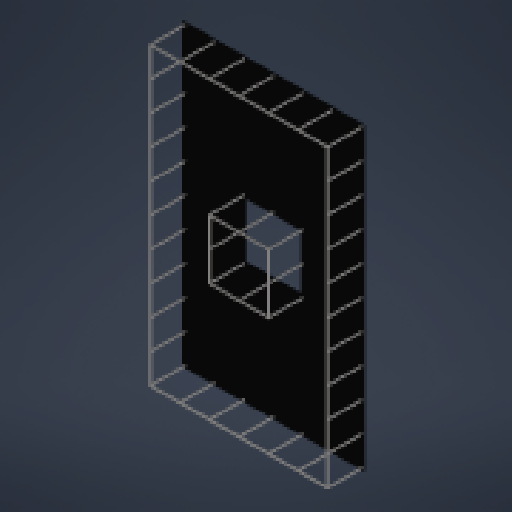
# Autodesk Inventor part: SecondFloor
Saved by Autodesk Inventor 2025 (Build 290162000, 162)
## iProperties
Created: 2024-05-05
Part Number: SecondFloor
Material: Generic
Document SubType Name: Modeling
Designer: zulet
Density: 1 g/cm^3
Appearance: Black
Author: zulet
Autodesk Inventor part; units mm, degrees
(part 1 of 2)
ref_plane "YZ Plane" through (0, 0, 0) normal (1, 0, 0) x (0, 1, 0)
ref_plane "XZ Plane" through (0, 0, 0) normal (0, 1, 0) x (-1, 0, 0)
ref_plane "XY Plane" through (0, 0, 0) normal (0, 0, 1) x (1, 0, 0)
sketch "Sketch1" plane through (0, 0, 0) normal (0, 0, 1) x (1, 0, 0)
  line L0 (183.513924, 6006.538309) -> (183.513924, 4506.538309)
  line L1 (183.513924, 7561.538309) -> (183.513924, 6006.538309)
  line L2 (183.513924, -48.461691) -> (183.513924, 1506.538309)
  line L3 (183.513924, 1506.538309) -> (183.513924, 3006.538309)
  line L4 (183.513924, 4506.538309) -> (183.513924, 3006.538309)
  line L5 (1738.513924, -48.461691) -> (183.513924, -48.461691)
  line L6 (3238.513924, -48.461691) -> (1738.513924, -48.461691)
  line L7 (3238.513924, -48.026006) -> (4793.513924, -48.026006)
  line L8 (4793.513924, -48.461691) -> (4793.513924, 1506.538309)
  line L9 (4793.513924, 3006.538309) -> (4793.513924, 1506.538309)
  line L10 (4793.513924, 3006.538309) -> (4793.513924, 4506.538309)
  line L11 (4793.513924, 4506.538309) -> (4793.513924, 6006.538309)
  line L12 (4793.513924, 7561.538309) -> (4793.513924, 6006.538309)
  line L13 (3238.513924, 7561.538309) -> (4793.513924, 7561.538309)
  line L14 (1738.513924, 7561.973994) -> (3238.513924, 7561.973994)
  line L15 (1738.513924, 7561.538309) -> (183.513924, 7561.538309)
  line L16 (3183.513924, 4561.538309) -> (1793.513924, 4561.538309)
  line L17 (1683.513924, 4451.538309) -> (1683.513924, 3061.538309)
  line L18 (3293.513924, 3061.538309) -> (3293.513924, 4451.538309)
  line L19 (1793.513924, 2951.538309) -> (3183.513924, 2951.538309)
  line L20 (3238.513924, 3006.538309) -> (3183.513924, 2951.538309)
  line L21 (3293.296081, 3061.756152) -> (3238.296081, 3006.756152)
  line L22 (3238.513924, 4506.538309) -> (3183.513924, 4561.538309)
  line L23 (3238.513924, 4506.538309) -> (3293.513924, 4451.538309)
  line L24 (1793.513924, 4561.538309) -> (1738.513924, 4506.538309)
  line L25 (1683.513924, 4451.538309) -> (1738.513924, 4506.538309)
  line L26 (1738.513924, 3006.538309) -> (1683.513924, 3061.538309)
  line L27 (1738.513924, 3006.538309) -> (1793.513924, 2951.538309)
  line L28 (3183.513924, 4451.538309) -> (1793.513924, 4451.538309)
  line L29 (1793.513924, 4451.538309) -> (1793.513924, 3061.538309)
  line L30 (3183.513924, 3061.538309) -> (3183.513924, 4451.538309)
  line L31 (1793.513924, 3061.538309) -> (3183.513924, 3061.538309)
  point P0 (0, 0)
  point P1 (1683.513924, 2185.44858)
  point P2 (1683.513924, 2831.394254)
sketch "Sketch1 outline for Extrusion1" plane through (0, 0, 0) normal (0, 0, 1) x (1, 0, 0)
  line L0 (1738.513924, 7561.538309) -> (183.513924, 7561.538309)
  line L1 (3238.513924, 7561.538309) -> (1738.513924, 7561.538309)
  line L2 (183.513924, 7561.538309) -> (183.513924, 6006.538309)
  line L3 (4793.513924, 7561.538309) -> (3238.513924, 7561.538309)
  line L4 (183.513924, 6006.538309) -> (183.513924, 4506.538309)
  line L5 (4793.513924, 6006.538309) -> (4793.513924, 7561.538309)
  line L6 (183.513924, 4506.538309) -> (183.513924, 3006.538309)
  line L7 (4793.513924, 4506.538309) -> (4793.513924, 6006.538309)
  line L8 (183.513924, 3006.538309) -> (183.513924, 1506.538309)
  line L9 (4793.513924, 3006.538309) -> (4793.513924, 4506.538309)
  line L10 (183.513924, 1506.538309) -> (183.513924, -48.461691)
  line L11 (4793.513924, 1506.538309) -> (4793.513924, 3006.538309)
  line L12 (183.513924, -48.461691) -> (1738.513924, -48.461691)
  line L13 (4793.513924, -48.461691) -> (4793.513924, 1506.538309)
  line L14 (1738.513924, -48.461691) -> (3238.513924, -48.461691)
  line L15 (3238.513924, -48.461691) -> (4793.513924, -48.461691)
  line L16 (3183.513924, 4451.538309) -> (3183.513924, 3061.538309)
  line L17 (1793.513924, 4451.538309) -> (3183.513924, 4451.538309)
  line L18 (1793.513924, 3061.538309) -> (1793.513924, 4451.538309)
  line L19 (3183.513924, 3061.538309) -> (1793.513924, 3061.538309)
extrude "Extrusion1" add sketch "Sketch1 outline for Extrusion1" along normal blind 20
sketch "Sketch2" plane through (0, 0, 20) normal (0, 0, 1) x (1, 0, 0)
  line L0 (231.513924, 7521.538309) -> (255.513924, 7521.538309)
  line L1 (263.513924, 7513.538309) -> (263.513924, 7489.538309)
  line L2 (255.513924, 7481.538309) -> (231.513924, 7481.538309)
  line L3 (223.513924, 7489.538309) -> (223.513924, 7513.538309)
  line L4 (4793.513924, 7561.538309) -> (183.513924, 7561.538309)
  line L5 (183.513924, 7561.538309) -> (183.513924, -48.461691)
  arc A0 (231.513924, 7521.538309) -> (223.513924, 7513.538309) centre (231.513924, 7513.538309) ccw
  arc A1 (263.513924, 7513.538309) -> (255.513924, 7521.538309) centre (255.513924, 7513.538309) ccw
  arc A2 (255.513924, 7481.538309) -> (263.513924, 7489.538309) centre (255.513924, 7489.538309) ccw
  arc A3 (223.513924, 7489.538309) -> (231.513924, 7481.538309) centre (231.513924, 7489.538309) ccw
  line L6 (981.513924, 7521.538309) -> (1005.513924, 7521.538309)
  line L7 (1013.513924, 7513.538309) -> (1013.513924, 7489.538309)
  line L8 (1005.513924, 7481.538309) -> (981.513924, 7481.538309)
  line L9 (973.513924, 7489.538309) -> (973.513924, 7513.538309)
  arc A4 (981.513924, 7521.538309) -> (973.513924, 7513.538309) centre (981.513924, 7513.538309) ccw
  arc A5 (1013.513924, 7513.538309) -> (1005.513924, 7521.538309) centre (1005.513924, 7513.538309) ccw
  arc A6 (1005.513924, 7481.538309) -> (1013.513924, 7489.538309) centre (1005.513924, 7489.538309) ccw
  arc A7 (973.513924, 7489.538309) -> (981.513924, 7481.538309) centre (981.513924, 7489.538309) ccw
  line L10 (1731.513924, 7521.538309) -> (1755.513924, 7521.538309)
  line L11 (1763.513924, 7513.538309) -> (1763.513924, 7489.538309)
  line L12 (1755.513924, 7481.538309) -> (1731.513924, 7481.538309)
  line L13 (1723.513924, 7489.538309) -> (1723.513924, 7513.538309)
  arc A8 (1731.513924, 7521.538309) -> (1723.513924, 7513.538309) centre (1731.513924, 7513.538309) ccw
  arc A9 (1763.513924, 7513.538309) -> (1755.513924, 7521.538309) centre (1755.513924, 7513.538309) ccw
  arc A10 (1755.513924, 7481.538309) -> (1763.513924, 7489.538309) centre (1755.513924, 7489.538309) ccw
  arc A11 (1723.513924, 7489.538309) -> (1731.513924, 7481.538309) centre (1731.513924, 7489.538309) ccw
  line L14 (2481.513924, 7521.538309) -> (2505.513924, 7521.538309)
  line L15 (2513.513924, 7513.538309) -> (2513.513924, 7489.538309)
  line L16 (2505.513924, 7481.538309) -> (2481.513924, 7481.538309)
  line L17 (2473.513924, 7489.538309) -> (2473.513924, 7513.538309)
  arc A12 (2481.513924, 7521.538309) -> (2473.513924, 7513.538309) centre (2481.513924, 7513.538309) ccw
  arc A13 (2513.513924, 7513.538309) -> (2505.513924, 7521.538309) centre (2505.513924, 7513.538309) ccw
  arc A14 (2505.513924, 7481.538309) -> (2513.513924, 7489.538309) centre (2505.513924, 7489.538309) ccw
  arc A15 (2473.513924, 7489.538309) -> (2481.513924, 7481.538309) centre (2481.513924, 7489.538309) ccw
  line L18 (3231.513924, 7521.538309) -> (3255.513924, 7521.538309)
  line L19 (3263.513924, 7513.538309) -> (3263.513924, 7489.538309)
  line L20 (3255.513924, 7481.538309) -> (3231.513924, 7481.538309)
  line L21 (3223.513924, 7489.538309) -> (3223.513924, 7513.538309)
  arc A16 (3231.513924, 7521.538309) -> (3223.513924, 7513.538309) centre (3231.513924, 7513.538309) ccw
  arc A17 (3263.513924, 7513.538309) -> (3255.513924, 7521.538309) centre (3255.513924, 7513.538309) ccw
  arc A18 (3255.513924, 7481.538309) -> (3263.513924, 7489.538309) centre (3255.513924, 7489.538309) ccw
  arc A19 (3223.513924, 7489.538309) -> (3231.513924, 7481.538309) centre (3231.513924, 7489.538309) ccw
  line L22 (3981.513924, 7521.538309) -> (4005.513924, 7521.538309)
  line L23 (4013.513924, 7513.538309) -> (4013.513924, 7489.538309)
  line L24 (4005.513924, 7481.538309) -> (3981.513924, 7481.538309)
  line L25 (3973.513924, 7489.538309) -> (3973.513924, 7513.538309)
  arc A20 (3981.513924, 7521.538309) -> (3973.513924, 7513.538309) centre (3981.513924, 7513.538309) ccw
  arc A21 (4013.513924, 7513.538309) -> (4005.513924, 7521.538309) centre (4005.513924, 7513.538309) ccw
  arc A22 (4005.513924, 7481.538309) -> (4013.513924, 7489.538309) centre (4005.513924, 7489.538309) ccw
  arc A23 (3973.513924, 7489.538309) -> (3981.513924, 7481.538309) centre (3981.513924, 7489.538309) ccw
  line L26 (4731.513924, 7521.538309) -> (4755.513924, 7521.538309)
  line L27 (4763.513924, 7513.538309) -> (4763.513924, 7489.538309)
  line L28 (4755.513924, 7481.538309) -> (4731.513924, 7481.538309)
  line L29 (4723.513924, 7489.538309) -> (4723.513924, 7513.538309)
  arc A24 (4731.513924, 7521.538309) -> (4723.513924, 7513.538309) centre (4731.513924, 7513.538309) ccw
  arc A25 (4763.513924, 7513.538309) -> (4755.513924, 7521.538309) centre (4755.513924, 7513.538309) ccw
  arc A26 (4755.513924, 7481.538309) -> (4763.513924, 7489.538309) centre (4755.513924, 7489.538309) ccw
  arc A27 (4723.513924, 7489.538309) -> (4731.513924, 7481.538309) centre (4731.513924, 7489.538309) ccw
  line L30 (231.513924, 6771.538309) -> (255.513924, 6771.538309)
  line L31 (263.513924, 6763.538309) -> (263.513924, 6739.538309)
  line L32 (255.513924, 6731.538309) -> (231.513924, 6731.538309)
  line L33 (223.513924, 6739.538309) -> (223.513924, 6763.538309)
  arc A28 (231.513924, 6771.538309) -> (223.513924, 6763.538309) centre (231.513924, 6763.538309) ccw
  arc A29 (263.513924, 6763.538309) -> (255.513924, 6771.538309) centre (255.513924, 6763.538309) ccw
  arc A30 (255.513924, 6731.538309) -> (263.513924, 6739.538309) centre (255.513924, 6739.538309) ccw
  arc A31 (223.513924, 6739.538309) -> (231.513924, 6731.538309) centre (231.513924, 6739.538309) ccw
  line L34 (981.513924, 6771.538309) -> (1005.513924, 6771.538309)
  line L35 (1013.513924, 6763.538309) -> (1013.513924, 6739.538309)
  line L36 (1005.513924, 6731.538309) -> (981.513924, 6731.538309)
  line L37 (973.513924, 6739.538309) -> (973.513924, 6763.538309)
  arc A32 (981.513924, 6771.538309) -> (973.513924, 6763.538309) centre (981.513924, 6763.538309) ccw
  arc A33 (1013.513924, 6763.538309) -> (1005.513924, 6771.538309) centre (1005.513924, 6763.538309) ccw
  arc A34 (1005.513924, 6731.538309) -> (1013.513924, 6739.538309) centre (1005.513924, 6739.538309) ccw
  arc A35 (973.513924, 6739.538309) -> (981.513924, 6731.538309) centre (981.513924, 6739.538309) ccw
  line L38 (1731.513924, 6771.538309) -> (1755.513924, 6771.538309)
  line L39 (1763.513924, 6763.538309) -> (1763.513924, 6739.538309)
  line L40 (1755.513924, 6731.538309) -> (1731.513924, 6731.538309)
  line L41 (1723.513924, 6739.538309) -> (1723.513924, 6763.538309)
  arc A36 (1731.513924, 6771.538309) -> (1723.513924, 6763.538309) centre (1731.513924, 6763.538309) ccw
  arc A37 (1763.513924, 6763.538309) -> (1755.513924, 6771.538309) centre (1755.513924, 6763.538309) ccw
  arc A38 (1755.513924, 6731.538309) -> (1763.513924, 6739.538309) centre (1755.513924, 6739.538309) ccw
  arc A39 (1723.513924, 6739.538309) -> (1731.513924, 6731.538309) centre (1731.513924, 6739.538309) ccw
  line L42 (2481.513924, 6771.538309) -> (2505.513924, 6771.538309)
  line L43 (2513.513924, 6763.538309) -> (2513.513924, 6739.538309)
  line L44 (2505.513924, 6731.538309) -> (2481.513924, 6731.538309)
  line L45 (2473.513924, 6739.538309) -> (2473.513924, 6763.538309)
  arc A40 (2481.513924, 6771.538309) -> (2473.513924, 6763.538309) centre (2481.513924, 6763.538309) ccw
  arc A41 (2513.513924, 6763.538309) -> (2505.513924, 6771.538309) centre (2505.513924, 6763.538309) ccw
  arc A42 (2505.513924, 6731.538309) -> (2513.513924, 6739.538309) centre (2505.513924, 6739.538309) ccw
  arc A43 (2473.513924, 6739.538309) -> (2481.513924, 6731.538309) centre (2481.513924, 6739.538309) ccw
  line L46 (3231.513924, 6771.538309) -> (3255.513924, 6771.538309)
  line L47 (3263.513924, 6763.538309) -> (3263.513924, 6739.538309)
  line L48 (3255.513924, 6731.538309) -> (3231.513924, 6731.538309)
  line L49 (3223.513924, 6739.538309) -> (3223.513924, 6763.538309)
  arc A44 (3231.513924, 6771.538309) -> (3223.513924, 6763.538309) centre (3231.513924, 6763.538309) ccw
  arc A45 (3263.513924, 6763.538309) -> (3255.513924, 6771.538309) centre (3255.513924, 6763.538309) ccw
  arc A46 (3255.513924, 6731.538309) -> (3263.513924, 6739.538309) centre (3255.513924, 6739.538309) ccw
  arc A47 (3223.513924, 6739.538309) -> (3231.513924, 6731.538309) centre (3231.513924, 6739.538309) ccw
  line L50 (3981.513924, 6771.538309) -> (4005.513924, 6771.538309)
  line L51 (4013.513924, 6763.538309) -> (4013.513924, 6739.538309)
  line L52 (4005.513924, 6731.538309) -> (3981.513924, 6731.538309)
  line L53 (3973.513924, 6739.538309) -> (3973.513924, 6763.538309)
  arc A48 (3981.513924, 6771.538309) -> (3973.513924, 6763.538309) centre (3981.513924, 6763.538309) ccw
  arc A49 (4013.513924, 6763.538309) -> (4005.513924, 6771.538309) centre (4005.513924, 6763.538309) ccw
  arc A50 (4005.513924, 6731.538309) -> (4013.513924, 6739.538309) centre (4005.513924, 6739.538309) ccw
  arc A51 (3973.513924, 6739.538309) -> (3981.513924, 6731.538309) centre (3981.513924, 6739.538309) ccw
  line L54 (4731.513924, 6771.538309) -> (4755.513924, 6771.538309)
  line L55 (4763.513924, 6763.538309) -> (4763.513924, 6739.538309)
  line L56 (4755.513924, 6731.538309) -> (4731.513924, 6731.538309)
  line L57 (4723.513924, 6739.538309) -> (4723.513924, 6763.538309)
  arc A52 (4731.513924, 6771.538309) -> (4723.513924, 6763.538309) centre (4731.513924, 6763.538309) ccw
  arc A53 (4763.513924, 6763.538309) -> (4755.513924, 6771.538309) centre (4755.513924, 6763.538309) ccw
  arc A54 (4755.513924, 6731.538309) -> (4763.513924, 6739.538309) centre (4755.513924, 6739.538309) ccw
  arc A55 (4723.513924, 6739.538309) -> (4731.513924, 6731.538309) centre (4731.513924, 6739.538309) ccw
  line L58 (231.513924, 6021.538309) -> (255.513924, 6021.538309)
  line L59 (263.513924, 6013.538309) -> (263.513924, 5989.538309)
  line L60 (255.513924, 5981.538309) -> (231.513924, 5981.538309)
  line L61 (223.513924, 5989.538309) -> (223.513924, 6013.538309)
  arc A56 (231.513924, 6021.538309) -> (223.513924, 6013.538309) centre (231.513924, 6013.538309) ccw
  arc A57 (263.513924, 6013.538309) -> (255.513924, 6021.538309) centre (255.513924, 6013.538309) ccw
  arc A58 (255.513924, 5981.538309) -> (263.513924, 5989.538309) centre (255.513924, 5989.538309) ccw
  arc A59 (223.513924, 5989.538309) -> (231.513924, 5981.538309) centre (231.513924, 5989.538309) ccw
  line L62 (981.513924, 6021.538309) -> (1005.513924, 6021.538309)
  line L63 (1013.513924, 6013.538309) -> (1013.513924, 5989.538309)
  line L64 (1005.513924, 5981.538309) -> (981.513924, 5981.538309)
  line L65 (973.513924, 5989.538309) -> (973.513924, 6013.538309)
  arc A60 (981.513924, 6021.538309) -> (973.513924, 6013.538309) centre (981.513924, 6013.538309) ccw
  arc A61 (1013.513924, 6013.538309) -> (1005.513924, 6021.538309) centre (1005.513924, 6013.538309) ccw
  arc A62 (1005.513924, 5981.538309) -> (1013.513924, 5989.538309) centre (1005.513924, 5989.538309) ccw
  arc A63 (973.513924, 5989.538309) -> (981.513924, 5981.538309) centre (981.513924, 5989.538309) ccw
  line L66 (1731.513924, 6021.538309) -> (1755.513924, 6021.538309)
  line L67 (1763.513924, 6013.538309) -> (1763.513924, 5989.538309)
  line L68 (1755.513924, 5981.538309) -> (1731.513924, 5981.538309)
  line L69 (1723.513924, 5989.538309) -> (1723.513924, 6013.538309)
  arc A64 (1731.513924, 6021.538309) -> (1723.513924, 6013.538309) centre (1731.513924, 6013.538309) ccw
  arc A65 (1763.513924, 6013.538309) -> (1755.513924, 6021.538309) centre (1755.513924, 6013.538309) ccw
  arc A66 (1755.513924, 5981.538309) -> (1763.513924, 5989.538309) centre (1755.513924, 5989.538309) ccw
  arc A67 (1723.513924, 5989.538309) -> (1731.513924, 5981.538309) centre (1731.513924, 5989.538309) ccw
  line L70 (2481.513924, 6021.538309) -> (2505.513924, 6021.538309)
  line L71 (2513.513924, 6013.538309) -> (2513.513924, 5989.538309)
  line L72 (2505.513924, 5981.538309) -> (2481.513924, 5981.538309)
  line L73 (2473.513924, 5989.538309) -> (2473.513924, 6013.538309)
  arc A68 (2481.513924, 6021.538309) -> (2473.513924, 6013.538309) centre (2481.513924, 6013.538309) ccw
  arc A69 (2513.513924, 6013.538309) -> (2505.513924, 6021.538309) centre (2505.513924, 6013.538309) ccw
  arc A70 (2505.513924, 5981.538309) -> (2513.513924, 5989.538309) centre (2505.513924, 5989.538309) ccw
  arc A71 (2473.513924, 5989.538309) -> (2481.513924, 5981.538309) centre (2481.513924, 5989.538309) ccw
  line L74 (3231.513924, 6021.538309) -> (3255.513924, 6021.538309)
  line L75 (3263.513924, 6013.538309) -> (3263.513924, 5989.538309)
  line L76 (3255.513924, 5981.538309) -> (3231.513924, 5981.538309)
  line L77 (3223.513924, 5989.538309) -> (3223.513924, 6013.538309)
  arc A72 (3231.513924, 6021.538309) -> (3223.513924, 6013.538309) centre (3231.513924, 6013.538309) ccw
  arc A73 (3263.513924, 6013.538309) -> (3255.513924, 6021.538309) centre (3255.513924, 6013.538309) ccw
  arc A74 (3255.513924, 5981.538309) -> (3263.513924, 5989.538309) centre (3255.513924, 5989.538309) ccw
  arc A75 (3223.513924, 5989.538309) -> (3231.513924, 5981.538309) centre (3231.513924, 5989.538309) ccw
  line L78 (3981.513924, 6021.538309) -> (4005.513924, 6021.538309)
  line L79 (4013.513924, 6013.538309) -> (4013.513924, 5989.538309)
  line L80 (4005.513924, 5981.538309) -> (3981.513924, 5981.538309)
  line L81 (3973.513924, 5989.538309) -> (3973.513924, 6013.538309)
  arc A76 (3981.513924, 6021.538309) -> (3973.513924, 6013.538309) centre (3981.513924, 6013.538309) ccw
  arc A77 (4013.513924, 6013.538309) -> (4005.513924, 6021.538309) centre (4005.513924, 6013.538309) ccw
  arc A78 (4005.513924, 5981.538309) -> (4013.513924, 5989.538309) centre (4005.513924, 5989.538309) ccw
  arc A79 (3973.513924, 5989.538309) -> (3981.513924, 5981.538309) centre (3981.513924, 5989.538309) ccw
  line L82 (4731.513924, 6021.538309) -> (4755.513924, 6021.538309)
  line L83 (4763.513924, 6013.538309) -> (4763.513924, 5989.538309)
  line L84 (4755.513924, 5981.538309) -> (4731.513924, 5981.538309)
  line L85 (4723.513924, 5989.538309) -> (4723.513924, 6013.538309)
  arc A80 (4731.513924, 6021.538309) -> (4723.513924, 6013.538309) centre (4731.513924, 6013.538309) ccw
  arc A81 (4763.513924, 6013.538309) -> (4755.513924, 6021.538309) centre (4755.513924, 6013.538309) ccw
  arc A82 (4755.513924, 5981.538309) -> (4763.513924, 5989.538309) centre (4755.513924, 5989.538309) ccw
  arc A83 (4723.513924, 5989.538309) -> (4731.513924, 5981.538309) centre (4731.513924, 5989.538309) ccw
  line L86 (231.513924, 5271.538309) -> (255.513924, 5271.538309)
  line L87 (263.513924, 5263.538309) -> (263.513924, 5239.538309)
  line L88 (255.513924, 5231.538309) -> (231.513924, 5231.538309)
  line L89 (223.513924, 5239.538309) -> (223.513924, 5263.538309)
  arc A84 (231.513924, 5271.538309) -> (223.513924, 5263.538309) centre (231.513924, 5263.538309) ccw
  arc A85 (263.513924, 5263.538309) -> (255.513924, 5271.538309) centre (255.513924, 5263.538309) ccw
  arc A86 (255.513924, 5231.538309) -> (263.513924, 5239.538309) centre (255.513924, 5239.538309) ccw
  arc A87 (223.513924, 5239.538309) -> (231.513924, 5231.538309) centre (231.513924, 5239.538309) ccw
  line L90 (981.513924, 5271.538309) -> (1005.513924, 5271.538309)
  line L91 (1013.513924, 5263.538309) -> (1013.513924, 5239.538309)
  line L92 (1005.513924, 5231.538309) -> (981.513924, 5231.538309)
  line L93 (973.513924, 5239.538309) -> (973.513924, 5263.538309)
  arc A88 (981.513924, 5271.538309) -> (973.513924, 5263.538309) centre (981.513924, 5263.538309) ccw
  arc A89 (1013.513924, 5263.538309) -> (1005.513924, 5271.538309) centre (1005.513924, 5263.538309) ccw
  arc A90 (1005.513924, 5231.538309) -> (1013.513924, 5239.538309) centre (1005.513924, 5239.538309) ccw
  arc A91 (973.513924, 5239.538309) -> (981.513924, 5231.538309) centre (981.513924, 5239.538309) ccw
  line L94 (1731.513924, 5271.538309) -> (1755.513924, 5271.538309)
  line L95 (1763.513924, 5263.538309) -> (1763.513924, 5239.538309)
  line L96 (1755.513924, 5231.538309) -> (1731.513924, 5231.538309)
  line L97 (1723.513924, 5239.538309) -> (1723.513924, 5263.538309)
  arc A92 (1731.513924, 5271.538309) -> (1723.513924, 5263.538309) centre (1731.513924, 5263.538309) ccw
  arc A93 (1763.513924, 5263.538309) -> (1755.513924, 5271.538309) centre (1755.513924, 5263.538309) ccw
  arc A94 (1755.513924, 5231.538309) -> (1763.513924, 5239.538309) centre (1755.513924, 5239.538309) ccw
  arc A95 (1723.513924, 5239.538309) -> (1731.513924, 5231.538309) centre (1731.513924, 5239.538309) ccw
  line L98 (2481.513924, 5271.538309) -> (2505.513924, 5271.538309)
  line L99 (2513.513924, 5263.538309) -> (2513.513924, 5239.538309)
  line L100 (2505.513924, 5231.538309) -> (2481.513924, 5231.538309)
  line L101 (2473.513924, 5239.538309) -> (2473.513924, 5263.538309)
  arc A96 (2481.513924, 5271.538309) -> (2473.513924, 5263.538309) centre (2481.513924, 5263.538309) ccw
  arc A97 (2513.513924, 5263.538309) -> (2505.513924, 5271.538309) centre (2505.513924, 5263.538309) ccw
  arc A98 (2505.513924, 5231.538309) -> (2513.513924, 5239.538309) centre (2505.513924, 5239.538309) ccw
  arc A99 (2473.513924, 5239.538309) -> (2481.513924, 5231.538309) centre (2481.513924, 5239.538309) ccw
  line L102 (3231.513924, 5271.538309) -> (3255.513924, 5271.538309)
  line L103 (3263.513924, 5263.538309) -> (3263.513924, 5239.538309)
  line L104 (3255.513924, 5231.538309) -> (3231.513924, 5231.538309)
  line L105 (3223.513924, 5239.538309) -> (3223.513924, 5263.538309)
  arc A100 (3231.513924, 5271.538309) -> (3223.513924, 5263.538309) centre (3231.513924, 5263.538309) ccw
  arc A101 (3263.513924, 5263.538309) -> (3255.513924, 5271.538309) centre (3255.513924, 5263.538309) ccw
  arc A102 (3255.513924, 5231.538309) -> (3263.513924, 5239.538309) centre (3255.513924, 5239.538309) ccw
  arc A103 (3223.513924, 5239.538309) -> (3231.513924, 5231.538309) centre (3231.513924, 5239.538309) ccw
  line L106 (3981.513924, 5271.538309) -> (4005.513924, 5271.538309)
  line L107 (4013.513924, 5263.538309) -> (4013.513924, 5239.538309)
  line L108 (4005.513924, 5231.538309) -> (3981.513924, 5231.538309)
  line L109 (3973.513924, 5239.538309) -> (3973.513924, 5263.538309)
  arc A104 (3981.513924, 5271.538309) -> (3973.513924, 5263.538309) centre (3981.513924, 5263.538309) ccw
  arc A105 (4013.513924, 5263.538309) -> (4005.513924, 5271.538309) centre (4005.513924, 5263.538309) ccw
  arc A106 (4005.513924, 5231.538309) -> (4013.513924, 5239.538309) centre (4005.513924, 5239.538309) ccw
  arc A107 (3973.513924, 5239.538309) -> (3981.513924, 5231.538309) centre (3981.513924, 5239.538309) ccw
  line L110 (4731.513924, 5271.538309) -> (4755.513924, 5271.538309)
  line L111 (4763.513924, 5263.538309) -> (4763.513924, 5239.538309)
  line L112 (4755.513924, 5231.538309) -> (4731.513924, 5231.538309)
  line L113 (4723.513924, 5239.538309) -> (4723.513924, 5263.538309)
  arc A108 (4731.513924, 5271.538309) -> (4723.513924, 5263.538309) centre (4731.513924, 5263.538309) ccw
  arc A109 (4763.513924, 5263.538309) -> (4755.513924, 5271.538309) centre (4755.513924, 5263.538309) ccw
  arc A110 (4755.513924, 5231.538309) -> (4763.513924, 5239.538309) centre (4755.513924, 5239.538309) ccw
  arc A111 (4723.513924, 5239.538309) -> (4731.513924, 5231.538309) centre (4731.513924, 5239.538309) ccw
  line L114 (231.513924, 4521.538309) -> (255.513924, 4521.538309)
  line L115 (263.513924, 4513.538309) -> (263.513924, 4489.538309)
  line L116 (255.513924, 4481.538309) -> (231.513924, 4481.538309)
  line L117 (223.513924, 4489.538309) -> (223.513924, 4513.538309)
  arc A112 (231.513924, 4521.538309) -> (223.513924, 4513.538309) centre (231.513924, 4513.538309) ccw
  arc A113 (263.513924, 4513.538309) -> (255.513924, 4521.538309) centre (255.513924, 4513.538309) ccw
  arc A114 (255.513924, 4481.538309) -> (263.513924, 4489.538309) centre (255.513924, 4489.538309) ccw
  arc A115 (223.513924, 4489.538309) -> (231.513924, 4481.538309) centre (231.513924, 4489.538309) ccw
  line L118 (981.513924, 4521.538309) -> (1005.513924, 4521.538309)
  line L119 (1013.513924, 4513.538309) -> (1013.513924, 4489.538309)
  line L120 (1005.513924, 4481.538309) -> (981.513924, 4481.538309)
  line L121 (973.513924, 4489.538309) -> (973.513924, 4513.538309)
  arc A116 (981.513924, 4521.538309) -> (973.513924, 4513.538309) centre (981.513924, 4513.538309) ccw
  arc A117 (1013.513924, 4513.538309) -> (1005.513924, 4521.538309) centre (1005.513924, 4513.538309) ccw
  arc A118 (1005.513924, 4481.538309) -> (1013.513924, 4489.538309) centre (1005.513924, 4489.538309) ccw
  arc A119 (973.513924, 4489.538309) -> (981.513924, 4481.538309) centre (981.513924, 4489.538309) ccw
  line L122 (1731.513924, 4521.538309) -> (1755.513924, 4521.538309)
  line L123 (1763.513924, 4513.538309) -> (1763.513924, 4489.538309)
  line L124 (1755.513924, 4481.538309) -> (1731.513924, 4481.538309)
  line L125 (1723.513924, 4489.538309) -> (1723.513924, 4513.538309)
  arc A120 (1731.513924, 4521.538309) -> (1723.513924, 4513.538309) centre (1731.513924, 4513.538309) ccw
  arc A121 (1763.513924, 4513.538309) -> (1755.513924, 4521.538309) centre (1755.513924, 4513.538309) ccw
  arc A122 (1755.513924, 4481.538309) -> (1763.513924, 4489.538309) centre (1755.513924, 4489.538309) ccw
  arc A123 (1723.513924, 4489.538309) -> (1731.513924, 4481.538309) centre (1731.513924, 4489.538309) ccw
  line L126 (2481.513924, 4521.538309) -> (2505.513924, 4521.538309)
  line L127 (2513.513924, 4513.538309) -> (2513.513924, 4489.538309)
  line L128 (2505.513924, 4481.538309) -> (2481.513924, 4481.538309)
  line L129 (2473.513924, 4489.538309) -> (2473.513924, 4513.538309)
  arc A124 (2481.513924, 4521.538309) -> (2473.513924, 4513.538309) centre (2481.513924, 4513.538309) ccw
  arc A125 (2513.513924, 4513.538309) -> (2505.513924, 4521.538309) centre (2505.513924, 4513.538309) ccw
  arc A126 (2505.513924, 4481.538309) -> (2513.513924, 4489.538309) centre (2505.513924, 4489.538309) ccw
  arc A127 (2473.513924, 4489.538309) -> (2481.513924, 4481.538309) centre (2481.513924, 4489.538309) ccw
  line L130 (3231.513924, 4521.538309) -> (3255.513924, 4521.538309)
  line L131 (3263.513924, 4513.538309) -> (3263.513924, 4489.538309)
  line L132 (3255.513924, 4481.538309) -> (3231.513924, 4481.538309)
  line L133 (3223.513924, 4489.538309) -> (3223.513924, 4513.538309)
  arc A128 (3231.513924, 4521.538309) -> (3223.513924, 4513.538309) centre (3231.513924, 4513.538309) ccw
  arc A129 (3263.513924, 4513.538309) -> (3255.513924, 4521.538309) centre (3255.513924, 4513.538309) ccw
  arc A130 (3255.513924, 4481.538309) -> (3263.513924, 4489.538309) centre (3255.513924, 4489.538309) ccw
  arc A131 (3223.513924, 4489.538309) -> (3231.513924, 4481.538309) centre (3231.513924, 4489.538309) ccw
  line L134 (3981.513924, 4521.538309) -> (4005.513924, 4521.538309)
  line L135 (4013.513924, 4513.538309) -> (4013.513924, 4489.538309)
  line L136 (4005.513924, 4481.538309) -> (3981.513924, 4481.538309)
  line L137 (3973.513924, 4489.538309) -> (3973.513924, 4513.538309)
  arc A132 (3981.513924, 4521.538309) -> (3973.513924, 4513.538309) centre (3981.513924, 4513.538309) ccw
  arc A133 (4013.513924, 4513.538309) -> (4005.513924, 4521.538309) centre (4005.513924, 4513.538309) ccw
  arc A134 (4005.513924, 4481.538309) -> (4013.513924, 4489.538309) centre (4005.513924, 4489.538309) ccw
  arc A135 (3973.513924, 4489.538309) -> (3981.513924, 4481.538309) centre (3981.513924, 4489.538309) ccw
  line L138 (4731.513924, 4521.538309) -> (4755.513924, 4521.538309)
  line L139 (4763.513924, 4513.538309) -> (4763.513924, 4489.538309)
  line L140 (4755.513924, 4481.538309) -> (4731.513924, 4481.538309)
  line L141 (4723.513924, 4489.538309) -> (4723.513924, 4513.538309)
  arc A136 (4731.513924, 4521.538309) -> (4723.513924, 4513.538309) centre (4731.513924, 4513.538309) ccw
  arc A137 (4763.513924, 4513.538309) -> (4755.513924, 4521.538309) centre (4755.513924, 4513.538309) ccw
  arc A138 (4755.513924, 4481.538309) -> (4763.513924, 4489.538309) centre (4755.513924, 4489.538309) ccw
  arc A139 (4723.513924, 4489.538309) -> (4731.513924, 4481.538309) centre (4731.513924, 4489.538309) ccw
  line L142 (231.513924, 3771.538309) -> (255.513924, 3771.538309)
  line L143 (263.513924, 3763.538309) -> (263.513924, 3739.538309)
  line L144 (255.513924, 3731.538309) -> (231.513924, 3731.538309)
  line L145 (223.513924, 3739.538309) -> (223.513924, 3763.538309)
  arc A140 (231.513924, 3771.538309) -> (223.513924, 3763.538309) centre (231.513924, 3763.538309) ccw
  arc A141 (263.513924, 3763.538309) -> (255.513924, 3771.538309) centre (255.513924, 3763.538309) ccw
  arc A142 (255.513924, 3731.538309) -> (263.513924, 3739.538309) centre (255.513924, 3739.538309) ccw
  arc A143 (223.513924, 3739.538309) -> (231.513924, 3731.538309) centre (231.513924, 3739.538309) ccw
  line L146 (981.513924, 3771.538309) -> (1005.513924, 3771.538309)
  line L147 (1013.513924, 3763.538309) -> (1013.513924, 3739.538309)
  line L148 (1005.513924, 3731.538309) -> (981.513924, 3731.538309)
  line L149 (973.513924, 3739.538309) -> (973.513924, 3763.538309)
  arc A144 (981.513924, 3771.538309) -> (973.513924, 3763.538309) centre (981.513924, 3763.538309) ccw
  arc A145 (1013.513924, 3763.538309) -> (1005.513924, 3771.538309) centre (1005.513924, 3763.538309) ccw
  arc A146 (1005.513924, 3731.538309) -> (1013.513924, 3739.538309) centre (1005.513924, 3739.538309) ccw
  arc A147 (973.513924, 3739.538309) -> (981.513924, 3731.538309) centre (981.513924, 3739.538309) ccw
  line L150 (1731.513924, 3771.538309) -> (1755.513924, 3771.538309)
  line L151 (1763.513924, 3763.538309) -> (1763.513924, 3739.538309)
  line L152 (1755.513924, 3731.538309) -> (1731.513924, 3731.538309)
  line L153 (1723.513924, 3739.538309) -> (1723.513924, 3763.538309)
  arc A148 (1731.513924, 3771.538309) -> (1723.513924, 3763.538309) centre (1731.513924, 3763.538309) ccw
  arc A149 (1763.513924, 3763.538309) -> (1755.513924, 3771.538309) centre (1755.513924, 3763.538309) ccw
  arc A150 (1755.513924, 3731.538309) -> (1763.513924, 3739.538309) centre (1755.513924, 3739.538309) ccw
  arc A151 (1723.513924, 3739.538309) -> (1731.513924, 3731.538309) centre (1731.513924, 3739.538309) ccw
  line L154 (2481.513924, 3771.538309) -> (2505.513924, 3771.538309)
  line L155 (2513.513924, 3763.538309) -> (2513.513924, 3739.538309)
  line L156 (2505.513924, 3731.538309) -> (2481.513924, 3731.538309)
  line L157 (2473.513924, 3739.538309) -> (2473.513924, 3763.538309)
  arc A152 (2481.513924, 3771.538309) -> (2473.513924, 3763.538309) centre (2481.513924, 3763.538309) ccw
  arc A153 (2513.513924, 3763.538309) -> (2505.513924, 3771.538309) centre (2505.513924, 3763.538309) ccw
  arc A154 (2505.513924, 3731.538309) -> (2513.513924, 3739.538309) centre (2505.513924, 3739.538309) ccw
  arc A155 (2473.513924, 3739.538309) -> (2481.513924, 3731.538309) centre (2481.513924, 3739.538309) ccw
  line L158 (3231.513924, 3771.538309) -> (3255.513924, 3771.538309)
  line L159 (3263.513924, 3763.538309) -> (3263.513924, 3739.538309)
  line L160 (3255.513924, 3731.538309) -> (3231.513924, 3731.538309)
  line L161 (3223.513924, 3739.538309) -> (3223.513924, 3763.538309)
  arc A156 (3231.513924, 3771.538309) -> (3223.513924, 3763.538309) centre (3231.513924, 3763.538309) ccw
  arc A157 (3263.513924, 3763.538309) -> (3255.513924, 3771.538309) centre (3255.513924, 3763.538309) ccw
  arc A158 (3255.513924, 3731.538309) -> (3263.513924, 3739.538309) centre (3255.513924, 3739.538309) ccw
  arc A159 (3223.513924, 3739.538309) -> (3231.513924, 3731.538309) centre (3231.513924, 3739.538309) ccw
  line L162 (3981.513924, 3771.538309) -> (4005.513924, 3771.538309)
  line L163 (4013.513924, 3763.538309) -> (4013.513924, 3739.538309)
  line L164 (4005.513924, 3731.538309) -> (3981.513924, 3731.538309)
  line L165 (3973.513924, 3739.538309) -> (3973.513924, 3763.538309)
  arc A160 (3981.513924, 3771.538309) -> (3973.513924, 3763.538309) centre (3981.513924, 3763.538309) ccw
  arc A161 (4013.513924, 3763.538309) -> (4005.513924, 3771.538309) centre (4005.513924, 3763.538309) ccw
  arc A162 (4005.513924, 3731.538309) -> (4013.513924, 3739.538309) centre (4005.513924, 3739.538309) ccw
  arc A163 (3973.513924, 3739.538309) -> (3981.513924, 3731.538309) centre (3981.513924, 3739.538309) ccw
  line L166 (4731.513924, 3771.538309) -> (4755.513924, 3771.538309)
  line L167 (4763.513924, 3763.538309) -> (4763.513924, 3739.538309)
  line L168 (4755.513924, 3731.538309) -> (4731.513924, 3731.538309)
  line L169 (4723.513924, 3739.538309) -> (4723.513924, 3763.538309)
  arc A164 (4731.513924, 3771.538309) -> (4723.513924, 3763.538309) centre (4731.513924, 3763.538309) ccw
  arc A165 (4763.513924, 3763.538309) -> (4755.513924, 3771.538309) centre (4755.513924, 3763.538309) ccw
  arc A166 (4755.513924, 3731.538309) -> (4763.513924, 3739.538309) centre (4755.513924, 3739.538309) ccw
  arc A167 (4723.513924, 3739.538309) -> (4731.513924, 3731.538309) centre (4731.513924, 3739.538309) ccw
  line L170 (231.513924, 3021.538309) -> (255.513924, 3021.538309)
  line L171 (263.513924, 3013.538309) -> (263.513924, 2989.538309)
  line L172 (255.513924, 2981.538309) -> (231.513924, 2981.538309)
  line L173 (223.513924, 2989.538309) -> (223.513924, 3013.538309)
  arc A168 (231.513924, 3021.538309) -> (223.513924, 3013.538309) centre (231.513924, 3013.538309) ccw
  arc A169 (263.513924, 3013.538309) -> (255.513924, 3021.538309) centre (255.513924, 3013.538309) ccw
  arc A170 (255.513924, 2981.538309) -> (263.513924, 2989.538309) centre (255.513924, 2989.538309) ccw
  arc A171 (223.513924, 2989.538309) -> (231.513924, 2981.538309) centre (231.513924, 2989.538309) ccw
  line L174 (981.513924, 3021.538309) -> (1005.513924, 3021.538309)
  line L175 (1013.513924, 3013.538309) -> (1013.513924, 2989.538309)
  line L176 (1005.513924, 2981.538309) -> (981.513924, 2981.538309)
  line L177 (973.513924, 2989.538309) -> (973.513924, 3013.538309)
  arc A172 (981.513924, 3021.538309) -> (973.513924, 3013.538309) centre (981.513924, 3013.538309) ccw
  arc A173 (1013.513924, 3013.538309) -> (1005.513924, 3021.538309) centre (1005.513924, 3013.538309) ccw
  arc A174 (1005.513924, 2981.538309) -> (1013.513924, 2989.538309) centre (1005.513924, 2989.538309) ccw
  arc A175 (973.513924, 2989.538309) -> (981.513924, 2981.538309) centre (981.513924, 2989.538309) ccw
  line L178 (1731.513924, 3021.538309) -> (1755.513924, 3021.538309)
  line L179 (1763.513924, 3013.538309) -> (1763.513924, 2989.538309)
  line L180 (1755.513924, 2981.538309) -> (1731.513924, 2981.538309)
  line L181 (1723.513924, 2989.538309) -> (1723.513924, 3013.538309)
  arc A176 (1731.513924, 3021.538309) -> (1723.513924, 3013.538309) centre (1731.513924, 3013.538309) ccw
  arc A177 (1763.513924, 3013.538309) -> (1755.513924, 3021.538309) centre (1755.513924, 3013.538309) ccw
  arc A178 (1755.513924, 2981.538309) -> (1763.513924, 2989.538309) centre (1755.513924, 2989.538309) ccw
  arc A179 (1723.513924, 2989.538309) -> (1731.513924, 2981.538309) centre (1731.513924, 2989.538309) ccw
  line L182 (2481.513924, 3021.538309) -> (2505.513924, 3021.538309)
  line L183 (2513.513924, 3013.538309) -> (2513.513924, 2989.538309)
  line L184 (2505.513924, 2981.538309) -> (2481.513924, 2981.538309)
  line L185 (2473.513924, 2989.538309) -> (2473.513924, 3013.538309)
  arc A180 (2481.513924, 3021.538309) -> (2473.513924, 3013.538309) centre (2481.513924, 3013.538309) ccw
  arc A181 (2513.513924, 3013.538309) -> (2505.513924, 3021.538309) centre (2505.513924, 3013.538309) ccw
  arc A182 (2505.513924, 2981.538309) -> (2513.513924, 2989.538309) centre (2505.513924, 2989.538309) ccw
  arc A183 (2473.513924, 2989.538309) -> (2481.513924, 2981.538309) centre (2481.513924, 2989.538309) ccw
  line L186 (3231.513924, 3021.538309) -> (3255.513924, 3021.538309)
  line L187 (3263.513924, 3013.538309) -> (3263.513924, 2989.538309)
  line L188 (3255.513924, 2981.538309) -> (3231.513924, 2981.538309)
  line L189 (3223.513924, 2989.538309) -> (3223.513924, 3013.538309)
  arc A184 (3231.513924, 3021.538309) -> (3223.513924, 3013.538309) centre (3231.513924, 3013.538309) ccw
  arc A185 (3263.513924, 3013.538309) -> (3255.513924, 3021.538309) centre (3255.513924, 3013.538309) ccw
  arc A186 (3255.513924, 2981.538309) -> (3263.513924, 2989.538309) centre (3255.513924, 2989.538309) ccw
  arc A187 (3223.513924, 2989.538309) -> (3231.513924, 2981.538309) centre (3231.513924, 2989.538309) ccw
  line L190 (3981.513924, 3021.538309) -> (4005.513924, 3021.538309)
  line L191 (4013.513924, 3013.538309) -> (4013.513924, 2989.538309)
  line L192 (4005.513924, 2981.538309) -> (3981.513924, 2981.538309)
  line L193 (3973.513924, 2989.538309) -> (3973.513924, 3013.538309)
  arc A188 (3981.513924, 3021.538309) -> (3973.513924, 3013.538309) centre (3981.513924, 3013.538309) ccw
  arc A189 (4013.513924, 3013.538309) -> (4005.513924, 3021.538309) centre (4005.513924, 3013.538309) ccw
  arc A190 (4005.513924, 2981.538309) -> (4013.513924, 2989.538309) centre (4005.513924, 2989.538309) ccw
  arc A191 (3973.513924, 2989.538309) -> (3981.513924, 2981.538309) centre (3981.513924, 2989.538309) ccw
  line L194 (4731.513924, 3021.538309) -> (4755.513924, 3021.538309)
  line L195 (4763.513924, 3013.538309) -> (4763.513924, 2989.538309)
  line L196 (4755.513924, 2981.538309) -> (4731.513924, 2981.538309)
  line L197 (4723.513924, 2989.538309) -> (4723.513924, 3013.538309)
  arc A192 (4731.513924, 3021.538309) -> (4723.513924, 3013.538309) centre (4731.513924, 3013.538309) ccw
  arc A193 (4763.513924, 3013.538309) -> (4755.513924, 3021.538309) centre (4755.513924, 3013.538309) ccw
  arc A194 (4755.513924, 2981.538309) -> (4763.513924, 2989.538309) centre (4755.513924, 2989.538309) ccw
  arc A195 (4723.513924, 2989.538309) -> (4731.513924, 2981.538309) centre (4731.513924, 2989.538309) ccw
  line L198 (231.513924, 2271.538309) -> (255.513924, 2271.538309)
  line L199 (263.513924, 2263.538309) -> (263.513924, 2239.538309)
  line L200 (255.513924, 2231.538309) -> (231.513924, 2231.538309)
  line L201 (223.513924, 2239.538309) -> (223.513924, 2263.538309)
  arc A196 (231.513924, 2271.538309) -> (223.513924, 2263.538309) centre (231.513924, 2263.538309) ccw
  arc A197 (263.513924, 2263.538309) -> (255.513924, 2271.538309) centre (255.513924, 2263.538309) ccw
  arc A198 (255.513924, 2231.538309) -> (263.513924, 2239.538309) centre (255.513924, 2239.538309) ccw
  arc A199 (223.513924, 2239.538309) -> (231.513924, 2231.538309) centre (231.513924, 2239.538309) ccw
  line L202 (981.513924, 2271.538309) -> (1005.513924, 2271.538309)
  line L203 (1013.513924, 2263.538309) -> (1013.513924, 2239.538309)
  line L204 (1005.513924, 2231.538309) -> (981.513924, 2231.538309)
  line L205 (973.513924, 2239.538309) -> (973.513924, 2263.538309)
  arc A200 (981.513924, 2271.538309) -> (973.513924, 2263.538309) centre (981.513924, 2263.538309) ccw
  arc A201 (1013.513924, 2263.538309) -> (1005.513924, 2271.538309) centre (1005.513924, 2263.538309) ccw
  arc A202 (1005.513924, 2231.538309) -> (1013.513924, 2239.538309) centre (1005.513924, 2239.538309) ccw
  arc A203 (973.513924, 2239.538309) -> (981.513924, 2231.538309) centre (981.513924, 2239.538309) ccw
  line L206 (1731.513924, 2271.538309) -> (1755.513924, 2271.538309)
  line L207 (1763.513924, 2263.538309) -> (1763.513924, 2239.538309)
  line L208 (1755.513924, 2231.538309) -> (1731.513924, 2231.538309)
  line L209 (1723.513924, 2239.538309) -> (1723.513924, 2263.538309)
  arc A204 (1731.513924, 2271.538309) -> (1723.513924, 2263.538309) centre (1731.513924, 2263.538309) ccw
  arc A205 (1763.513924, 2263.538309) -> (1755.513924, 2271.538309) centre (1755.513924, 2263.538309) ccw
  arc A206 (1755.513924, 2231.538309) -> (1763.513924, 2239.538309) centre (1755.513924, 2239.538309) ccw
  arc A207 (1723.513924, 2239.538309) -> (1731.513924, 2231.538309) centre (1731.513924, 2239.538309) ccw
  line L210 (2481.513924, 2271.538309) -> (2505.513924, 2271.538309)
  line L211 (2513.513924, 2263.538309) -> (2513.513924, 2239.538309)
  line L212 (2505.513924, 2231.538309) -> (2481.513924, 2231.538309)
  line L213 (2473.513924, 2239.538309) -> (2473.513924, 2263.538309)
  arc A208 (2481.513924, 2271.538309) -> (2473.513924, 2263.538309) centre (2481.513924, 2263.538309) ccw
  arc A209 (2513.513924, 2263.538309) -> (2505.513924, 2271.538309) centre (2505.513924, 2263.538309) ccw
  arc A210 (2505.513924, 2231.538309) -> (2513.513924, 2239.538309) centre (2505.513924, 2239.538309) ccw
  arc A211 (2473.513924, 2239.538309) -> (2481.513924, 2231.538309) centre (2481.513924, 2239.538309) ccw
  line L214 (3231.513924, 2271.538309) -> (3255.513924, 2271.538309)
  line L215 (3263.513924, 2263.538309) -> (3263.513924, 2239.538309)
  line L216 (3255.513924, 2231.538309) -> (3231.513924, 2231.538309)
  line L217 (3223.513924, 2239.538309) -> (3223.513924, 2263.538309)
  arc A212 (3231.513924, 2271.538309) -> (3223.513924, 2263.538309) centre (3231.513924, 2263.538309) ccw
  arc A213 (3263.513924, 2263.538309) -> (3255.513924, 2271.538309) centre (3255.513924, 2263.538309) ccw
  arc A214 (3255.513924, 2231.538309) -> (3263.513924, 2239.538309) centre (3255.513924, 2239.538309) ccw
  arc A215 (3223.513924, 2239.538309) -> (3231.513924, 2231.538309) centre (3231.513924, 2239.538309) ccw
  line L218 (3981.513924, 2271.538309) -> (4005.513924, 2271.538309)
  line L219 (4013.513924, 2263.538309) -> (4013.513924, 2239.538309)
  line L220 (4005.513924, 2231.538309) -> (3981.513924, 2231.538309)
  line L221 (3973.513924, 2239.538309) -> (3973.513924, 2263.538309)
  arc A216 (3981.513924, 2271.538309) -> (3973.513924, 2263.538309) centre (3981.513924, 2263.538309) ccw
  arc A217 (4013.513924, 2263.538309) -> (4005.513924, 2271.538309) centre (4005.513924, 2263.538309) ccw
  arc A218 (4005.513924, 2231.538309) -> (4013.513924, 2239.538309) centre (4005.513924, 2239.538309) ccw
  arc A219 (3973.513924, 2239.538309) -> (3981.513924, 2231.538309) centre (3981.513924, 2239.538309) ccw
  line L222 (4731.513924, 2271.538309) -> (4755.513924, 2271.538309)
  line L223 (4763.513924, 2263.538309) -> (4763.513924, 2239.538309)
  line L224 (4755.513924, 2231.538309) -> (4731.513924, 2231.538309)
  line L225 (4723.513924, 2239.538309) -> (4723.513924, 2263.538309)
  arc A220 (4731.513924, 2271.538309) -> (4723.513924, 2263.538309) centre (4731.513924, 2263.538309) ccw
  arc A221 (4763.513924, 2263.538309) -> (4755.513924, 2271.538309) centre (4755.513924, 2263.538309) ccw
  arc A222 (4755.513924, 2231.538309) -> (4763.513924, 2239.538309) centre (4755.513924, 2239.538309) ccw
  arc A223 (4723.513924, 2239.538309) -> (4731.513924, 2231.538309) centre (4731.513924, 2239.538309) ccw
  line L226 (231.513924, 1521.538309) -> (255.513924, 1521.538309)
  line L227 (263.513924, 1513.538309) -> (263.513924, 1489.538309)
  line L228 (255.513924, 1481.538309) -> (231.513924, 1481.538309)
  line L229 (223.513924, 1489.538309) -> (223.513924, 1513.538309)
  arc A224 (231.513924, 1521.538309) -> (223.513924, 1513.538309) centre (231.513924, 1513.538309) ccw
  arc A225 (263.513924, 1513.538309) -> (255.513924, 1521.538309) centre (255.513924, 1513.538309) ccw
  arc A226 (255.513924, 1481.538309) -> (263.513924, 1489.538309) centre (255.513924, 1489.538309) ccw
  arc A227 (223.513924, 1489.538309) -> (231.513924, 1481.538309) centre (231.513924, 1489.538309) ccw
  line L230 (981.513924, 1521.538309) -> (1005.513924, 1521.538309)
  line L231 (1013.513924, 1513.538309) -> (1013.513924, 1489.538309)
  line L232 (1005.513924, 1481.538309) -> (981.513924, 1481.538309)
  line L233 (973.513924, 1489.538309) -> (973.513924, 1513.538309)
  arc A228 (981.513924, 1521.538309) -> (973.513924, 1513.538309) centre (981.513924, 1513.538309) ccw
  arc A229 (1013.513924, 1513.538309) -> (1005.513924, 1521.538309) centre (1005.513924, 1513.538309) ccw
  arc A230 (1005.513924, 1481.538309) -> (1013.513924, 1489.538309) centre (1005.513924, 1489.538309) ccw
  arc A231 (973.513924, 1489.538309) -> (981.513924, 1481.538309) centre (981.513924, 1489.538309) ccw
  line L234 (1731.513924, 1521.538309) -> (1755.513924, 1521.538309)
  line L235 (1763.513924, 1513.538309) -> (1763.513924, 1489.538309)
  line L236 (1755.513924, 1481.538309) -> (1731.513924, 1481.538309)
  line L237 (1723.513924, 1489.538309) -> (1723.513924, 1513.538309)
  arc A232 (1731.513924, 1521.538309) -> (1723.513924, 1513.538309) centre (1731.513924, 1513.538309) ccw
  arc A233 (1763.513924, 1513.538309) -> (1755.513924, 1521.538309) centre (1755.513924, 1513.538309) ccw
  arc A234 (1755.513924, 1481.538309) -> (1763.513924, 1489.538309) centre (1755.513924, 1489.538309) ccw
  arc A235 (1723.513924, 1489.538309) -> (1731.513924, 1481.538309) centre (1731.513924, 1489.538309) ccw
  line L238 (2481.513924, 1521.538309) -> (2505.513924, 1521.538309)
  line L239 (2513.513924, 1513.538309) -> (2513.513924, 1489.538309)
  line L240 (2505.513924, 1481.538309) -> (2481.513924, 1481.538309)
  line L241 (2473.513924, 1489.538309) -> (2473.513924, 1513.538309)
  arc A236 (2481.513924, 1521.538309) -> (2473.513924, 1513.538309) centre (2481.513924, 1513.538309) ccw
  arc A237 (2513.513924, 1513.538309) -> (2505.513924, 1521.538309) centre (2505.513924, 1513.538309) ccw
  arc A238 (2505.513924, 1481.538309) -> (2513.513924, 1489.538309) centre (2505.513924, 1489.538309) ccw
  arc A239 (2473.513924, 1489.538309) -> (2481.513924, 1481.538309) centre (2481.513924, 1489.538309) ccw
  line L242 (3231.513924, 1521.538309) -> (3255.513924, 1521.538309)
  line L243 (3263.513924, 1513.538309) -> (3263.513924, 1489.538309)
  line L244 (3255.513924, 1481.538309) -> (3231.513924, 1481.538309)
  line L245 (3223.513924, 1489.538309) -> (3223.513924, 1513.538309)
  arc A240 (3231.513924, 1521.538309) -> (3223.513924, 1513.538309) centre (3231.513924, 1513.538309) ccw
  arc A241 (3263.513924, 1513.538309) -> (3255.513924, 1521.538309) centre (3255.513924, 1513.538309) ccw
  arc A242 (3255.513924, 1481.538309) -> (3263.513924, 1489.538309) centre (3255.513924, 1489.538309) ccw
  arc A243 (3223.513924, 1489.538309) -> (3231.513924, 1481.538309) centre (3231.513924, 1489.538309) ccw
  line L246 (3981.513924, 1521.538309) -> (4005.513924, 1521.538309)
  line L247 (4013.513924, 1513.538309) -> (4013.513924, 1489.538309)
  line L248 (4005.513924, 1481.538309) -> (3981.513924, 1481.538309)
  line L249 (3973.513924, 1489.538309) -> (3973.513924, 1513.538309)
  arc A244 (3981.513924, 1521.538309) -> (3973.513924, 1513.538309) centre (3981.513924, 1513.538309) ccw
  arc A245 (4013.513924, 1513.538309) -> (4005.513924, 1521.538309) centre (4005.513924, 1513.538309) ccw
  arc A246 (4005.513924, 1481.538309) -> (4013.513924, 1489.538309) centre (4005.513924, 1489.538309) ccw
  arc A247 (3973.513924, 1489.538309) -> (3981.513924, 1481.538309) centre (3981.513924, 1489.538309) ccw
  line L250 (4731.513924, 1521.538309) -> (4755.513924, 1521.538309)
  line L251 (4763.513924, 1513.538309) -> (4763.513924, 1489.538309)
  line L252 (4755.513924, 1481.538309) -> (4731.513924, 1481.538309)
  line L253 (4723.513924, 1489.538309) -> (4723.513924, 1513.538309)
  arc A248 (4731.513924, 1521.538309) -> (4723.513924, 1513.538309) centre (4731.513924, 1513.538309) ccw
  arc A249 (4763.513924, 1513.538309) -> (4755.513924, 1521.538309) centre (4755.513924, 1513.538309) ccw
  arc A250 (4755.513924, 1481.538309) -> (4763.513924, 1489.538309) centre (4755.513924, 1489.538309) ccw
  arc A251 (4723.513924, 1489.538309) -> (4731.513924, 1481.538309) centre (4731.513924, 1489.538309) ccw
  line L254 (231.513924, 771.538309) -> (255.513924, 771.538309)
  line L255 (263.513924, 763.538309) -> (263.513924, 739.538309)
  line L256 (255.513924, 731.538309) -> (231.513924, 731.538309)
  line L257 (223.513924, 739.538309) -> (223.513924, 763.538309)
  arc A252 (231.513924, 771.538309) -> (223.513924, 763.538309) centre (231.513924, 763.538309) ccw
  arc A253 (263.513924, 763.538309) -> (255.513924, 771.538309) centre (255.513924, 763.538309) ccw
  arc A254 (255.513924, 731.538309) -> (263.513924, 739.538309) centre (255.513924, 739.538309) ccw
  arc A255 (223.513924, 739.538309) -> (231.513924, 731.538309) centre (231.513924, 739.538309) ccw
  line L258 (981.513924, 771.538309) -> (1005.513924, 771.538309)
  line L259 (1013.513924, 763.538309) -> (1013.513924, 739.538309)
  line L260 (1005.513924, 731.538309) -> (981.513924, 731.538309)
  line L261 (973.513924, 739.538309) -> (973.513924, 763.538309)
  arc A256 (981.513924, 771.538309) -> (973.513924, 763.538309) centre (981.513924, 763.538309) ccw
  arc A257 (1013.513924, 763.538309) -> (1005.513924, 771.538309) centre (1005.513924, 763.538309) ccw
  arc A258 (1005.513924, 731.538309) -> (1013.513924, 739.538309) centre (1005.513924, 739.538309) ccw
  arc A259 (973.513924, 739.538309) -> (981.513924, 731.538309) centre (981.513924, 739.538309) ccw
  line L262 (1731.513924, 771.538309) -> (1755.513924, 771.538309)
  line L263 (1763.513924, 763.538309) -> (1763.513924, 739.538309)
  line L264 (1755.513924, 731.538309) -> (1731.513924, 731.538309)
  line L265 (1723.513924, 739.538309) -> (1723.513924, 763.538309)
  arc A260 (1731.513924, 771.538309) -> (1723.513924, 763.538309) centre (1731.513924, 763.538309) ccw